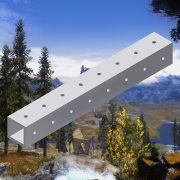
# Autodesk Inventor part: C28_TK_FrontWheelGuard
Saved by Autodesk Inventor 2015 SP1 (Build 190203100, 203)
## iProperties
Created: 2016-01-29
Part Number: C28_TK_FrontWheelGuard
Material: Aluminum 6061
Document SubType Name: Modeling
Designer: TheeTimatahee
Density: 2.7 g/cm^3
Appearance: Aluminum - Flat
Mass: 151.165 g
Surface Area: 371.534 cm^2
Volume: 55.9869 cm^3
Author: TheeTimatahee
Autodesk Inventor part; units mm, degrees
ref_plane "YZ Plane" through (0, 0, 0) normal (1, 0, 0) x (0, 1, 0)
ref_plane "XZ Plane" through (0, 0, 0) normal (0, 1, 0) x (-1, 0, 0)
ref_plane "XY Plane" through (0, 0, 0) normal (0, 0, 1) x (1, 0, 0)
sketch "Sketch1" plane through (0, 0, 0) normal (0, 0, 1) x (1, 0, 0)
  line L0 (-12.7, -12.7) -> (12.7, -12.7)
  line L1 (12.7, -12.7) -> (12.7, 12.7)
  line L2 (12.7, 12.7) -> (-12.7, 12.7)
  line L3 (-12.7, 12.7) -> (-12.7, -12.7)
  line L4 (-12.7, -12.7) -> (12.7, 12.7) construction
  line L5 (12.7, -12.7) -> (-12.7, 12.7) construction
  line L6 (9.525, -9.525) -> (-9.525, -9.525)
  line L7 (-9.525, -9.525) -> (-9.525, 9.525)
  line L8 (-9.525, 9.525) -> (9.525, 9.525)
  line L9 (9.525, 9.525) -> (9.525, -9.525)
  line L10 (9.525, -9.525) -> (-9.525, 9.525) construction
  line L11 (-9.525, -9.525) -> (9.525, 9.525) construction
  point P0 (0, 0)
  dimension "d0" = 25.4
  dimension "d1" = 25.4
  dimension "d6" = 3.175
  dimension "d7" = 3.175
  constraints: 24 end point, 4 midpoint, 4 parallel, 2 horizontal, 2 perpendicular
  measures "d0" distance of L2.end L1.end
  measures "d1" distance of L0.end L1.end
  measures "d6" distance between parallel lines of L2 L8
  measures "d7" distance between parallel lines of L3 L7
extrude "Extrusion1" add sketch "Sketch1" along normal blind 203.2
sketch "Sketch6" plane through (12.7, -12.7, 0) normal (1, 0, 0) x (0, 0, -1)
  line L0 (0, 0) -> (0, 25.4) projected
  line L1 (0, 25.4) -> (-203.2, 25.4) projected
  point P0 (0, 12.7)
  point P1 (-12.7, 12.7)
  point P2 (-38.1, 12.7)
  point P3 (-63.5, 12.7)
  point P4 (-88.9, 12.7)
  point P5 (-114.3, 12.7)
  point P6 (-139.7, 12.7)
  point P7 (-165.1, 12.7)
  point P8 (-190.5, 12.7)
  dimension "d23" = 12.7
  dimension "d24" = 12.7
  dimension "d27" = 25.4
  constraints: 1 horizontal, 7 other
  measures "d23" distance from line of L0 point (-12.7, 12.7)
  measures "d24" distance from line of L1 point (-12.7, 12.7)
  measures "d27" distance of point (-12.7, 12.7) point (-38.1, 12.7)
hole "Hole2" at (12.7, 0, 12.7) at (12.7, 0, 38.1) at (12.7, 0, 63.5) at (12.7, 0, 88.9) at (12.7, 0, 114.3) at (12.7, 0, 139.7) at (12.7, 0, 165.1) at (12.7, 0, 190.5) direction (-1, 0, 0) diameter 4.1402 end through all
sketch "Sketch7" plane through (-12.7, 12.7, 0) normal (0, 1, 0) x (1, 0, 0)
  line L0 (25.4, 0) -> (0, 0) projected
  line L1 (0, 0) -> (0, -203.2) projected
  point P0 (12.7, 0)
  point P1 (12.7, -12.7)
  point P2 (12.7, -38.1)
  point P3 (12.7, -63.5)
  point P4 (12.7, -88.9)
  point P5 (12.7, -114.3)
  point P6 (12.7, -139.7)
  point P7 (12.7, -165.1)
  point P8 (12.7, -190.5)
  dimension "d39" = 12.7
  dimension "d40" = 12.7
  dimension "d43" = 25.4
  constraints: 1 vertical, 7 other
  measures "d39" distance from line of L0 point (12.7, -12.7)
  measures "d40" distance from line of L1 point (12.7, -12.7)
  measures "d43" distance of point (12.7, -12.7) point (12.7, -38.1)
hole "Hole3" at (0, 12.7, 12.7) at (0, 12.7, 38.1) at (0, 12.7, 63.5) at (0, 12.7, 88.9) at (0, 12.7, 114.3) at (0, 12.7, 139.7) at (0, 12.7, 165.1) at (0, 12.7, 190.5) direction (0, -1, 0) diameter 4.1402 end through all
body "Solid1"
